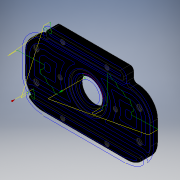
# Autodesk Inventor part: Ball Shifter plate
Saved by Autodesk Inventor 2018.3 (Build 223284000, 284)
## iProperties
Created: 2019-12-16
Part Number: Ball Shifter plate
Material: Aluminum 6061
Document SubType Name: Modeling
Designer: kedri
Density: 2.7 g/cm^3
Appearance: Anodized - Black
Mass: 102.417 g
Surface Area: 154.461 cm^2
Volume: 37.9324 cm^3
Author: kedri
Autodesk Inventor part; units mm, degrees
ref_plane "YZ Plane" through (0, 0, 0) normal (1, 0, 0) x (0, 1, 0)
ref_plane "XZ Plane" through (0, 0, 0) normal (0, 1, 0) x (-1, 0, 0)
ref_plane "XY Plane" through (0, 0, 0) normal (0, 0, 1) x (1, 0, 0)
sketch "Sketch1" plane through (0, 0, 0) normal (0, 0, 1) x (1, 0, 0)
  line L0 (0, 0) -> (107.95, 0)
  line L1 (107.95, 0) -> (107.95, 63.5)
  line L2 (107.95, 63.5) -> (0, 63.5)
  line L3 (0, 63.5) -> (0, 0)
  circle A0 centre (53.975, 30.226) radius 11.1125
  point P0 (9.525, 16.129)
  point P1 (9.525, 41.529)
  point P2 (98.425, 41.529)
  point P3 (98.425, 16.129)
  dimension "d0" = 107.95
  dimension "d1" = 63.5
  dimension "d2" = 22.225
  dimension "d3" = 30.226
  dimension "d4" = 53.975
  dimension "d5" = 16.129
  dimension "d7" = 21.971
  dimension "d53" = 44.45
  dimension "d54" = 44.45
  dimension "d55" = 25.4
  constraints: 8 end point, 2 horizontal alignment, 2 parallel, 2 vertical alignment, 1 centre point, 1 horizontal, 1 perpendicular
  measures "d0" distance of L2.end L1.end
  measures "d1" distance of L1.end L0.end
  measures "d2" diameter of A0
  measures "d3" distance from line of L0 A0.centre
  measures "d4" distance from line of L1 A0.centre
  measures "d5" distance from line of L0 point (9.525, 16.129)
  measures "d7" distance from line of L2 point (9.525, 41.529)
  measures "d53" horizontal distance of A0.centre point (9.525, 41.529)
  measures "d54" horizontal distance of A0.centre point (98.425, 41.529)
  measures "d55" distance of point (9.525, 16.129) point (9.525, 41.529)
extrude "Extrusion1" add sketch "Sketch1" against normal blind 6.35
hole "Hole1" at (9.525, 16.129, 0) at (9.525, 41.529, 0) at (98.425, 41.529, 0) at (98.425, 16.129, 0) direction (0, 0, -1) diameter 4.9784 end through all thread size "1/4-20 UNC" class "2B" standard "ANSI Unified Screw Threads"
sketch "Sketch2" plane through (107.95, 0, 0) normal (1, 0, 0) x (0, 0, -1)
  line L0 (0, 0) -> (-2.54, 0)
  line L1 (-2.54, 0) -> (-2.54, 6.35)
  line L2 (-2.54, 6.35) -> (0, 6.35)
  line L3 (0, 6.35) -> (0, 0)
  line L4 (0, 63.5) -> (0, 0) projected
  line L5 (0, 63.5) -> (-2.54, 63.5)
  line L6 (-2.54, 63.5) -> (-2.54, 57.15)
  line L7 (-2.54, 57.15) -> (0, 57.15)
  line L8 (0, 57.15) -> (0, 63.5)
  dimension "d18" = 2.54
  dimension "d19" = 6.35
  dimension "d20" = 2.54
  dimension "d21" = 6.35
  constraints: 16 end point, 4 parallel, 2 horizontal, 2 perpendicular
  measures "d18" distance of L1.end L2.end
  measures "d19" distance of L0.end L1.end
  measures "d20" distance of L7.end L6.end
  measures "d21" distance of L6.end L5.end
extrude "Extrusion2" add sketch "Sketch2" against normal up to surface (107.95 mm away)
sketch "Sketch3" plane through (0, 0, -6.35) normal (0, 0, -1) x (-1, 0, 0)
  line L0 (-107.95, 63.5) -> (-87.3125, 63.5)
  line L1 (-87.3125, 63.5) -> (-87.3125, 52.3875)
  line L2 (-87.3125, 52.3875) -> (-107.95, 52.3875)
  line L3 (-107.95, 52.3875) -> (-107.95, 63.5)
  line L4 (0, 0) -> (0, 63.5) projected
  line L5 (0, 63.5) -> (-20.6375, 63.5)
  line L6 (-20.6375, 63.5) -> (-20.6375, 52.3875)
  line L7 (-20.6375, 52.3875) -> (0, 52.3875)
  line L8 (0, 52.3875) -> (0, 63.5)
  dimension "d24" = 20.6375
  dimension "d25" = 11.1125
  dimension "d26" = 20.6375
  dimension "d27" = 11.1125
  constraints: 16 end point, 4 parallel, 2 horizontal, 2 perpendicular
  measures "d24" distance of L1.end L2.end
  measures "d25" distance of L0.end L1.end
  measures "d26" distance of L7.end L6.end
  measures "d27" distance of L5.end L6.end
extrude "Extrusion3" cut sketch "Sketch3" against normal up to surface (8.89 mm away)
fillet "Fillet1" radius 17.4625 4 edges at (0, 0, -1.905) (107.95, 0, -1.905) (107.95, 52.3875, -3.175) (0, 52.3875, -3.175)
fillet "Fillet3" radius 3.175 4 edges at (87.3125, 52.3875, -3.175) (20.6375, 52.3875, -3.175) (87.3125, 63.5, -1.905) (20.6375, 63.5, -1.905)
sketch "Sketch4" plane through (20.6375, 57.15, 2.54) normal (0, 0, 1) x (1, 0, 0)
  circle A0 centre (33.3375, -26.924) radius 11.1125 projected
  line L0 (66.675, 0) -> (0, 0) projected
  line L1 (83.3204, -50.8) -> (-16.6454, -50.8) projected
  point P0 (-20.6375, -57.15)
  point P1 (14.2875, 3.1242)
  point P2 (52.3875, 3.1242)
  point P3 (14.2875, -53.9242)
  point P4 (52.3875, -53.9242)
  dimension "d33" = 19.05
  dimension "d34" = 19.05
  dimension "d35" = 3.1242
  dimension "d36" = 3.1242
  constraints: 2 horizontal alignment, 2 vertical alignment
  measures "d33" horizontal distance of A0.centre point (14.287, 3.124)
  measures "d34" horizontal distance of A0.centre point (52.388, 3.124)
  measures "d35" distance from line of L0 point (14.287, 3.124)
  measures "d36" distance from line of L1 point (14.288, -53.924)
hole "Hole2" at (34.925, 60.2742, 2.54) at (73.025, 60.2742, 2.54) at (34.925, 3.2258, 2.54) at (73.025, 3.2258, 2.54) direction (0, 0, -1) diameter 3.9624 end through all thread size "10-32 UNF" class "2B" standard "ANSI Unified Screw Threads"
sketch "Sketch5" plane through (0, 0, 0) normal (0, 0, 1) x (1, 0, 0)
  circle A0 centre (53.975, 30.226) radius 11.1125 projected
  point P0 (0, 0)
  point P1 (30.1625, 30.226)
  point P2 (77.7875, 30.226)
  dimension "d44" = 23.8125
  dimension "d45" = 23.8125
  constraints: 2 horizontal alignment
  measures "d44" distance of A0.centre point (30.162, 30.226)
  measures "d45" distance of A0.centre point (77.788, 30.226)
hole "Hole3" at (30.1625, 30.226, 0) at (77.7875, 30.226, 0) direction (0, 0, -1) diameter 3.9624 end through all thread size "10-32 UNF" class "2B" standard "ANSI Unified Screw Threads"
fillet "Fillet4" radius 1.27 4 edges at (103.9579, 6.35, 1.27) (3.9921, 6.35, 1.27) (87.3125, 57.15, 1.27) (20.6375, 57.15, 1.27)
sketch "Sketch7" plane through (0, 0, 0) normal (0, 0, 1) x (1, 0, 0)
  circle A0 centre (53.975, 30.226) radius 11.1125 projected
  circle A1 centre (53.975, 30.226) radius 15.875
  point P0 (0, 0)
  dimension "d58" = 31.75
  constraints: 1 centre point, 1 coincident
  measures "d58" diameter of A1
extrude "Extrusion4" cut sketch "Sketch7" against normal blind 1.6002
equation "\"d4\" = 0.5 * d0"
equation "\"d54\" = d53"
equation "\"d20\" = d18"
equation "\"d34\" = d33"
equation "\"d45\" = d44"
body "Solid1"
